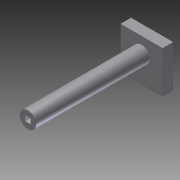
# Autodesk Inventor part: linac arm2
Saved by Autodesk Inventor 2011 (Build 150239000, 239)
## iProperties
Created: 2011-10-08
Part Number: linac arm2
Document SubType Name: Modeling
Designer: Matthew
Density: 1 g/cm^3
Author: Matthew
Autodesk Inventor part; units mm, degrees
ref_plane "YZ Plane" through (0, 0, 0) normal (1, 0, 0) x (0, 1, 0)
ref_plane "XZ Plane" through (0, 0, 0) normal (0, 1, 0) x (-1, 0, 0)
ref_plane "XY Plane" through (0, 0, 0) normal (0, 0, 1) x (1, 0, 0)
sketch "Sketch1" plane through (0, 0, 0) normal (0, 0, 1) x (1, 0, 0)
  circle A0 centre (0, 0) radius 9.906
  dimension "d0" = 19.812
  constraints: 1 centre point, 1 coincident
  measures "d0" diameter of A0
extrude "Extrusion1" add sketch "Sketch1" along normal blind 149.86
sketch "Sketch2" plane through (0, 0, 149.86) normal (0, 0, 1) x (1, 0, 0)
  circle A0 centre (0, 0) radius 9.906 projected
  circle A1 centre (0, 0) radius 3.175
  line L0 (-3.175, 0) -> (0, 0)
  line L1 (0, 0) -> (0, 3.175)
  line L2 (0, 3.175) -> (-3.175, 3.175)
  line L3 (-3.175, 3.175) -> (-3.175, 0)
  line L4 (-3.175, 3.175) -> (3.175, 3.175)
  line L5 (3.175, 3.175) -> (3.175, -3.175)
  line L6 (3.175, -3.175) -> (-3.175, -3.175)
  line L7 (-3.175, -3.175) -> (-3.175, 3.175)
  dimension "d3" = 6.35
  constraints: 16 end point, 4 parallel, 2 horizontal, 2 perpendicular, 2 point on circle, 1 centre point, 1 coincident
  measures "d3" diameter of A1
extrude "Extrusion2" cut sketch "Sketch2" against normal blind 12.7 contours A1 L0 L1 | L5 L6 A1 | A1 L4 L5 | L1 L0 A1 | A1 L3 L2 | L6 L7 A1
sketch "Sketch3" plane through (0, 0, 0) normal (0, 0, -1) x (-1, 0, 0)
  circle A0 centre (0, 0) radius 9.906 projected
  line L0 (0, 0) -> (-25.4, 0)
  line L1 (-25.4, 0) -> (-25.4, 25.4)
  line L2 (-25.4, 25.4) -> (0, 25.4)
  line L3 (0, 25.4) -> (0, 0)
  line L4 (-25.4, 25.4) -> (25.4, 25.4)
  line L5 (25.4, 25.4) -> (25.4, -25.4)
  line L6 (25.4, -25.4) -> (-25.4, -25.4)
  line L7 (-25.4, -25.4) -> (-25.4, 25.4)
  dimension "d6" = 25.4
  dimension "d7" = 25.4
  dimension "d8" = 50.8
  dimension "d9" = 50.8
  constraints: 16 end point, 4 parallel, 2 horizontal, 2 perpendicular
  measures "d6" distance of L1.end L2.end
  measures "d7" distance of L0.end L1.end
  measures "d8" distance of L5.end L6.end
  measures "d9" distance of L4.end L5.end
extrude "Extrusion3" add sketch "Sketch3" against normal blind 12.7 contours A0 L3 L4 L5 L6 L7 L0 | L3 L0 A0 | A0 L0 L1 L2 L3 picked at (-6.1942, 2.1674)
sketch "Sketch4" plane through (-25.4, 25.4, 0) normal (0, 1, 0) x (1, 0, 0)
  line L0 (0, -12.7) -> (50.8, -12.7) projected
  line L1 (50.8, 0) -> (50.8, -12.7) projected
  line L2 (0, 0) -> (50.8, 0) projected
  line L3 (0, 0) -> (0, -12.7) projected
  point P0 (25.4, 0)
extrude "Extrusion4" cut sketch "Sketch4" against normal blind 6.35
sketch "Sketch5" plane through (0, 0, 0) normal (0, 0, -1) x (-1, 0, 0)
  line L0 (25.4, 19.05) -> (-25.4, 19.05) projected
  line L1 (-25.4, 19.05) -> (-25.4, -25.4) projected
  line L2 (-25.4, -25.4) -> (25.4, -25.4) projected
  line L3 (25.4, -25.4) -> (25.4, 19.05) projected
  line L4 (-25.4, 19.05) -> (25.4, 19.05)
  line L5 (25.4, 19.05) -> (25.4, -31.75)
  line L6 (25.4, -31.75) -> (-25.4, -31.75)
  line L7 (-25.4, -31.75) -> (-25.4, 19.05)
  point P0 (0, 0)
  dimension "d14" = 50.8
  constraints: 8 end point, 2 parallel, 1 horizontal, 1 perpendicular
  measures "d14" distance of L4.end L5.end
extrude "Extrusion5" add sketch "Sketch5" against normal blind 12.7 contours L5 L6 L7 L2
sketch "Sketch7" plane through (0, 0, 12.7) normal (0, 0, 1) x (1, 0, 0)
  line L0 (25.4, 19.05) -> (25.4, -31.75) projected
  circle A0 centre (0, 0) radius 9.906 projected
  line L1 (0, 9.906) -> (0, 16.6116)
  line L2 (0, 16.6116) -> (-19.7866, 16.6116)
  line L3 (-19.7866, 16.6116) -> (-19.7866, -57.277)
  line L4 (-19.7866, -57.277) -> (0, -57.277)
  line L5 (0, -57.277) -> (0, 16.6116)
  line L6 (-19.7866, 16.6116) -> (19.7866, 16.6116)
  line L7 (19.7866, 16.6116) -> (19.7866, -57.277)
  line L8 (19.7866, -57.277) -> (-19.7866, -57.277)
  line L9 (-19.7866, -57.277) -> (-19.7866, 16.6116)
  dimension "d17" = 6.7056
  dimension "d18" = 19.7866
  dimension "d19" = 73.8886
  dimension "d20" = 39.5732
  constraints: 18 end point, 5 parallel, 2 horizontal, 2 perpendicular, 1 vertical alignment, 1 other
  measures "d17" distance of L1.start L1.end
  measures "d18" distance of L4.end L3.end
  measures "d19" distance of L3.end L2.end
  measures "d20" distance of L7.end L8.end
extrude "Extrusion6" add sketch "Sketch7" against normal blind 50.8 contours A0 L1 L6 L7 L8 L5 | L5 A0 | A0 L5 L4 L3 L2 L1 picked at (-4.6219, 0.7927)
sketch "Sketch8" plane through (0, 0, 0) normal (0, 0, -1) x (-1, 0, 0)
  line L0 (-19.7866, -31.75) -> (-19.7866, 16.6116) projected
  line L1 (-19.7866, 16.6116) -> (19.7866, 16.6116) projected
  line L2 (19.7866, 16.6116) -> (19.7866, -31.75) projected
  line L3 (19.7866, -31.75) -> (25.4, -31.75) projected
  line L4 (25.4, -31.75) -> (25.4, 19.05) projected
  line L5 (25.4, 19.05) -> (-25.4, 19.05) projected
  line L6 (-25.4, 19.05) -> (-25.4, -31.75) projected
  line L7 (-25.4, -31.75) -> (-19.7866, -31.75) projected
  point P0 (0, 0)
extrude "Extrusion7" cut sketch "Sketch8" against normal blind 50.8
fillet "Fillet1" radius 6.35 4 edges at (19.7866, 16.6116, -12.7) (-19.7866, 16.6116, -12.7) (19.7866, -57.277, -12.7) (-19.7866, -57.277, -12.7)
sketch "Sketch9" plane through (0, 0, -38.1) normal (0, 0, -1) x (-1, 0, 0)
  arc A0 (13.4366, -57.277) -> (19.7866, -50.927) centre (13.4366, -50.927) ccw projected
  line L0 (19.7866, 10.2616) -> (19.7866, -50.927) projected
  arc A1 (19.7866, 10.2616) -> (13.4366, 16.6116) centre (13.4366, 10.2616) ccw projected
  line L1 (-13.4366, 16.6116) -> (13.4366, 16.6116) projected
  arc A2 (-13.4366, 16.6116) -> (-19.7866, 10.2616) centre (-13.4366, 10.2616) ccw projected
  line L2 (-19.7866, -50.927) -> (-19.7866, 10.2616) projected
  arc A3 (-19.7866, -50.927) -> (-13.4366, -57.277) centre (-13.4366, -50.927) ccw projected
  line L3 (13.4366, -57.277) -> (-13.4366, -57.277) projected
  line L4 (0, -9.906) -> (0, 9.906) projected
  arc A4 (0, 9.906) -> (0, -9.906) centre (0, 0) ccw projected
extrude "Extrusion8" cut sketch "Sketch9" against normal blind 25.4
sketch "Sketch10" plane through (0, 0, -12.7) normal (0, 0, -1) x (-1, 0, 0)
  arc A0 (0, 9.906) -> (0, -9.906) centre (0, 0) ccw projected
  line L0 (0, -9.906) -> (0, 9.906) projected
extrude "Extrusion9" add sketch "Sketch10" against normal blind 25.4
sketch "Sketch11" plane through (0, 0, -12.7) normal (0, 0, -1) x (-1, 0, 0)
  line L0 (19.7866, 10.2616) -> (19.7866, -50.927) projected
  arc A0 (19.7866, 10.2616) -> (13.4366, 16.6116) centre (13.4366, 10.2616) ccw projected
  line L1 (-13.4366, 16.6116) -> (13.4366, 16.6116) projected
  arc A1 (-13.4366, 16.6116) -> (-19.7866, 10.2616) centre (-13.4366, 10.2616) ccw projected
  line L2 (-19.7866, -50.927) -> (-19.7866, 10.2616) projected
  arc A2 (-19.7866, -50.927) -> (-13.4366, -57.277) centre (-13.4366, -50.927) ccw projected
  line L3 (13.4366, -57.277) -> (-13.4366, -57.277) projected
  arc A3 (13.4366, -57.277) -> (19.7866, -50.927) centre (13.4366, -50.927) ccw projected
  point P0 (0, 0)
extrude "Extrusion10" cut sketch "Sketch11" against normal blind 12.7
sketch "Sketch12" plane through (0, 0, 0) normal (0, 0, -1) x (-1, 0, 0)
  line L0 (-19.7866, 16.6116) -> (19.7866, 16.6116)
  line L1 (19.7866, 16.6116) -> (19.7866, -57.277)
  line L2 (19.7866, -57.277) -> (-19.7866, -57.277)
  line L3 (-19.7866, -57.277) -> (-19.7866, 16.6116)
  point P0 (0, 0)
  constraints: 8 end point, 2 parallel, 1 horizontal, 1 perpendicular
extrude "Extrusion11" add sketch "Sketch12" against normal blind 12.7
fillet "Fillet2" radius 7.62 4 edges at (19.7866, 16.6116, 6.35) (-19.7866, 16.6116, 6.35) (-19.7866, -57.277, 6.35) (19.7866, -57.277, 6.35)
sketch "Sketch13" plane through (0, 0, 0) normal (0, 0, -1) x (-1, 0, 0)
  arc A0 (-19.7866, -49.657) -> (-12.1666, -57.277) centre (-12.1666, -49.657) ccw projected
  line L0 (12.1666, -57.277) -> (-12.1666, -57.277) projected
  arc A1 (12.1666, -57.277) -> (19.7866, -49.657) centre (12.1666, -49.657) ccw projected
  line L1 (19.7866, 8.9916) -> (19.7866, -49.657) projected
  arc A2 (19.7866, 8.9916) -> (12.1666, 16.6116) centre (12.1666, 8.9916) ccw projected
  line L2 (-12.1666, 16.6116) -> (12.1666, 16.6116) projected
  arc A3 (-12.1666, 16.6116) -> (-19.7866, 8.9916) centre (-12.1666, 8.9916) ccw projected
  line L3 (-19.7866, -49.657) -> (-19.7866, 8.9916) projected
  arc A4 (18.8199, 8.9916) -> (12.1666, 15.6449) centre (12.1666, 8.9916) ccw
  line L4 (18.8199, 8.9916) -> (18.8199, -49.657)
  arc A5 (12.1666, -56.3103) -> (18.8199, -49.657) centre (12.1666, -49.657) ccw
  line L5 (12.1666, -56.3103) -> (-12.1666, -56.3103)
  arc A6 (-18.8199, -49.657) -> (-12.1666, -56.3103) centre (-12.1666, -49.657) ccw
  line L6 (-18.8199, -49.657) -> (-18.8199, 8.9916)
  arc A7 (-12.1666, 15.6449) -> (-18.8199, 8.9916) centre (-12.1666, 8.9916) ccw
  line L7 (-12.1666, 15.6449) -> (12.1666, 15.6449)
  point P0 (0, 0)
  constraints: 8 end point, 8 point on circle, 4 centre point, 7 other
extrude "Extrusion12" cut sketch "Sketch13" against normal blind 12.7
sketch "Sketch14" plane through (0, 0, 0) normal (0, 0, -1) x (-1, 0, 0)
  line L0 (12.1666, 15.6449) -> (-12.1666, 15.6449) projected
  arc A0 (-12.1666, 15.6449) -> (-18.8199, 8.9916) centre (-12.1666, 8.9916) ccw projected
  line L1 (-18.8199, 8.9916) -> (-18.8199, -49.657) projected
  arc A1 (-18.8199, -49.657) -> (-12.1666, -56.3103) centre (-12.1666, -49.657) ccw projected
  line L2 (-12.1666, -56.3103) -> (12.1666, -56.3103) projected
  arc A2 (12.1666, -56.3103) -> (18.8199, -49.657) centre (12.1666, -49.657) ccw projected
  line L3 (18.8199, -49.657) -> (18.8199, 8.9916) projected
  arc A3 (18.8199, 8.9916) -> (12.1666, 15.6449) centre (12.1666, 8.9916) ccw projected
  point P0 (0, 0)
extrude "Extrusion13" cut sketch "Sketch14" against normal blind 2.54
sketch "Sketch15" plane through (0, 0, 2.54) normal (0, 0, -1) x (-1, 0, 0)
  arc A0 (-12.1666, 15.6449) -> (-18.8199, 8.9916) centre (-12.1666, 8.9916) ccw projected
  line L0 (-18.8199, -49.657) -> (-18.8199, 8.9916) projected
  arc A1 (-18.8199, -49.657) -> (-12.1666, -56.3103) centre (-12.1666, -49.657) ccw projected
  line L1 (12.1666, -56.3103) -> (-12.1666, -56.3103) projected
  arc A2 (12.1666, -56.3103) -> (18.8199, -49.657) centre (12.1666, -49.657) ccw projected
  line L2 (18.8199, 8.9916) -> (18.8199, -49.657) projected
  arc A3 (18.8199, 8.9916) -> (12.1666, 15.6449) centre (12.1666, 8.9916) ccw projected
  line L3 (-12.1666, 15.6449) -> (12.1666, 15.6449) projected
  point P0 (0, 0)
body "Solid1"
